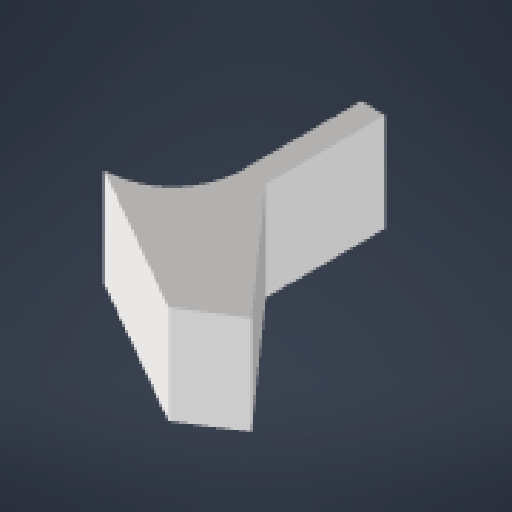
# Autodesk Inventor part: shock_absorber_holder
Saved by Autodesk Inventor 2024 (Build 280153000, 153)
## iProperties
Created: 2023-11-15
Part Number: shock_absorber_holder
Material: Типовые
Document SubType Name: Modeling
Designer: user
Density: 1 g/cm^3
Appearance: По умолчанию
Author: user
Autodesk Inventor part; units mm, degrees
ref_plane "YZ Plane" through (0, 0, 0) normal (1, 0, 0) x (0, 1, 0)
ref_plane "XZ Plane" through (0, 0, 0) normal (0, 1, 0) x (-1, 0, 0)
ref_plane "XY Plane" through (0, 0, 0) normal (0, 0, 1) x (1, 0, 0)
sketch "Эскиз1" plane through (0, 0, 0) normal (0, 0, 1) x (1, 0, 0)
  arc A0 (-10, -10) -> (10, 10) centre (-10, 10) ccw projected
  line L0 (-10, -10) -> (10, -10) construction
  line L1 (10, -10) -> (10, 25) construction
  line L2 (10, -10) -> (-120, -10) construction
  line L3 (10, 45) -> (10, 25) construction
  line L4 (10, 10) -> (10, 45)
  line L5 (10, 45) -> (15, 45)
  line L6 (15, 45) -> (15, 10)
  arc A1 (29.1975, -60) -> (42.8088, -40) centre (35, -49.3173) ccw
  arc A2 (-10, -10) -> (29.1975, -60) centre (67.3818, 10.299) ccw
  arc A3 (15, 10) -> (42.8088, -40) centre (94.196, 21.3136) ccw
  circle A4 centre (35, -49.3173) radius 1.5
  point P0 (0, 0)
  dimension "d6" = 5
  dimension "d7" = 20
  dimension "d8" = 80
  dimension "d9" = 25
  dimension "d10" = 80
  dimension "d11" = 50
  dimension "d15" = 3
  constraints: 6 end point, 6 point on circle, 4 centre point, 3 tangent, 1 coincident, 1 collinear, 1 horizontal, 1 horizontal alignment, 1 perpendicular
  measures "d6" distance of L5.end L3.start
  measures "d7" vertical distance of A1.end A1.start
  measures "d8" radius of A2
  measures "d9" horizontal distance of A1.centre L0.end
  measures "d10" radius of A3
  measures "d11" vertical distance of A1.end L6.end
  measures "d15" diameter of A4
extrude "Выдавливание1" add sketch "Эскиз1" along normal blind 28.75
ref_plane "РабПлоскость2" through (47.1569, -49.3173, 0) normal (1, 0, 0) x (0, 0, -1)
sketch "Эскиз4" plane through (47.1569, -49.3173, 0) normal (1, 0, 0) x (0, 0, -1)
  line L0 (0, -12.1569) -> (-28.75, -12.1569) construction
  line L1 (0, 9.3173) -> (-28.75, 9.3173) construction
  line L2 (-12.15, -12.1569) -> (-19.85, -12.1569)
  line L3 (-19.85, -12.1569) -> (-19.85, 9.3173)
  line L4 (-19.85, 9.3173) -> (-12.15, 9.3173)
  line L5 (-12.15, 9.3173) -> (-12.15, -12.1569)
  line L6 (-12.15, 124.4543) -> (-12.15, 113.7772) construction
  line L7 (-19.85, 113.7772) -> (-19.85, 124.4543) construction
  point P0 (0, 49.3173)
  constraints: 8 end point, 2 parallel, 2 point on line, 2 vertical alignment, 1 horizontal, 1 perpendicular
extrude "Выдавливание4" cut sketch "Эскиз4" against normal blind 85
fillet "Сопряжение1" radius 15 1 edges at (42.8088, -40, 16)
sketch "Эскиз6" plane through (0, 0, 0) normal (0, 0, -1) x (-1, 0, 0)
  circle A0 centre (-35, -49.3173) radius 1.5 construction
  line L0 (-32.6184, -50.6923) -> (-35, -52.0673)
  line L1 (-35, -52.0673) -> (-37.3816, -50.6923)
  line L2 (-37.3816, -50.6923) -> (-37.3816, -47.9423)
  line L3 (-37.3816, -47.9423) -> (-35, -46.5673)
  line L4 (-35, -46.5673) -> (-32.6184, -47.9423)
  line L5 (-32.6184, -47.9423) -> (-32.6184, -50.6923)
  point P0 (0, 0)
  dimension "d16" = 5.5
  constraints: 12 end point, 1 coincident, 1 vertical, 13 other
  measures "d16" distance of L0.end L3.end
extrude "Выдавливание5" cut sketch "Эскиз6" against normal blind 9
sketch "Эскиз7" plane through (0, 0, 0) normal (0, 0, -1) x (-1, 0, 0)
  arc A0 (-29.1975, -60) -> (10, -10) centre (-67.3818, 10.299) ccw construction
  line L0 (-10, -10) -> (120, -10) construction
  line L1 (10, -10) -> (28.8386, -10)
  line L2 (28.8386, -10) -> (28.8386, -14)
  line L3 (28.8386, -14) -> (8.8386, -14)
  arc A1 (8.8386, -14) -> (10, -10) centre (-67.3818, 10.299) ccw
  point P0 (0, 0)
  dimension "d19" = 4
  dimension "d20" = 20
  constraints: 6 end point, 3 point on circle, 1 centre point, 1 concentric, 1 perpendicular, 1 point on line, 1 vertical
  measures "d19" distance of L1.end L2.end
  measures "d20" distance of L2.end L3.end
extrude "Выдавливание6" add sketch "Эскиз7" against normal up to surface (28.75 mm away)
sketch "Эскиз8" plane through (-28.8386, -14, 0) normal (0, -1, 0) x (1, 0, 0)
  circle A0 centre (9.4193, 14.375) radius 2
  line L0 (20, 28.75) -> (20, 0) projected
  line L1 (0, 0) -> (18.8386, 0) projected
  point P0 (28.8386, 0)
  point P1 (20, 14.375)
  point P2 (9.4193, 0)
  dimension "d25" = 4
  constraints: 2 midpoint, 1 centre point, 1 horizontal alignment, 1 vertical alignment
  measures "d25" diameter of A0
extrude "Выдавливание7" cut sketch "Эскиз8" against normal blind 14.25
fillet "Сопряжение2" radius 15 2 edges at (-28.8386, -12, 0) (-28.8386, -12, 28.75)
sketch "Эскиз9" plane through (15, 10, 0) normal (1, 0, 0) x (0, 0, -1)
  line L0 (20, 15) -> (-170, 15) construction
  line L1 (20, 35) -> (-170, 35) construction
  line L2 (-28.75, 0) -> (-28.75, 35) construction
  line L3 (0, 0) -> (0, 35) construction
  circle A0 centre (-8.375, 25) radius 2
  circle A1 centre (-20.375, 25) radius 2
  line L4 (0, 35) -> (-28.75, 35) construction
  line L5 (0, 15) -> (0, 35) construction
  line L6 (-8.375, 25) -> (-20.375, 25) construction
  line L7 (0, 0) -> (-28.75, 0) construction
  line L8 (0, 0) -> (-28.75, 0) construction
  point P0 (0, -10)
  point P1 (0, 25)
  point P2 (-14.375, 0)
  point P3 (-14.375, 25)
  dimension "d27" = 4
  dimension "d28" = 12
  constraints: 6 end point, 3 midpoint, 2 centre point, 2 horizontal, 2 horizontal alignment, 2 point on line, 1 equal radius, 1 vertical, 1 vertical alignment
  measures "d27" diameter of A0
  measures "d28" distance of L6.start L6.end
extrude "Выдавливание8" cut sketch "Эскиз9" against normal blind 14.25
fillet "Сопряжение3" radius 15 2 edges at (12.5, 45, 28.75) (12.5, 45, 0)
chamfer "Фаска1" distance 9 distance2 3 3 edges at (45.0502, -56.1571, 12.15) (16.1986, -51.1849, 12.15) (32.5597, -29.686, 12.15) measured on face at (32.1745, -30.0048, 12.15) measured on face at (44.6368, -55.8758, 12.15) measured on face at (16.5185, -50.8006, 12.15)
chamfer "Фаска2" distance 9 distance2 3 3 edges at (45.0502, -56.1571, 19.85) (32.5597, -29.686, 19.85) (16.1986, -51.1849, 19.85) measured on face at (32.1745, -30.0048, 19.85) measured on face at (44.6368, -55.8758, 19.85) measured on face at (16.5185, -50.8006, 19.85)
